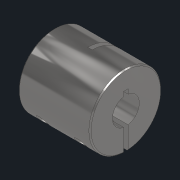
# Autodesk Inventor part: D_CPRC16-6-6
Saved by Autodesk Inventor 2022 (Build 260153000, 153)
## iProperties
Part Number: D_CPRC16-6-6
Material: 鋼、炭素鋼
Catalog Web Link: www.cadenas.de
Description: D_CPRC, CPRSC-Couplings - Rigid, Clamping Type
Vendor: MISUMI
Document SubType Name: Modeling
Designer: partserver
Manufacturer: MISUMI
Mass: 18.6575 g
Surface Area: 18.8292 cm^2
Volume: 2.37676 cm^3
Density: 7.85 g/cm^3
Appearance: 半つや出し
Category: PARTsolutions
Company: MISUMI
PSOL_IDENT_0: {$CADENAS_DATA\23d-libs\misumi\metric\50_couplings\parts\cprc.prj},182 {VTYP=3D},{NB=D_CPRC16-6-6},{
PSOL_IDENT_1: LINA=D_CPRC16-6-6},{NN=D_CPRC, CPRSC},{DATE=30.06.2021 13:25:02},{GEOMDATE=15.01.2008 11:35:00},{VER
PSOL_IDENT_2: SION=},{LINEID=10},{WBVAR=MAT,DD1,DD2},{WBNUMERIC=}  {NB=D_CPRC16-6-6},{LINA=D_CPRC16-6-6},{KT=DUMMY
PSOL_IDENT_3: },{PN=CPRC16-6-6},{MAT=1},{MATALG='1','Aluminium Alloy','2','Stainless Steel'},{ST=Alumite},{AC=Hex
PSOL_IDENT_4: Socket Head Cap Screw},{TYPE=CPRC},{D=16},{DD1=6},{DD1ALG1='5','5','6','6'},{DL=6},{DD2=6},{DD2ALG1='
PSOL_IDENT_5: 6','6'},{DR=6},{L=16},{M=2.5},{TSI=M2.5},{A=5},{A1=5.000},{TT=1},{TT1=1.000},{F=3.75},{TTT=1},{AT=0.
PSOL_IDENT_6: 3},{F1=3.750},{TSI1=4.800},{SC1=2.500},{SC2=5.970},{TSMD=2.500},{TSMIN=2.013},{L6=4.000}
NB: D_CPRC16-6-6
NN: D_CPRC, CPRSC
NT: Couplings - Rigid, Clamping Type
NBSYN: D_$TYPE.$D.-$DD1.-$DD2.
LINA: D_CPRC16-6-6
CATALOG: Misumi
PN: CPRC16-6-6
MAT: Aluminium Alloy
ST: Alumite
AC: Hex Socket Head Cap Screw
D: 16
DD1: 6
DD2: 6
L: 16
M: 2.5
A: 5
TT: 1
F: 3.75
SUPPLIER: MISUMI
ARTICLENO: D_CPRC16-6-6
BOMINFO: D_CPRC16-6-6
CREATOR: CADENAS GmbH
Title: D_CPRC16-6-6
Author: Cadenas PARTsolutions
Comments: Couplings - Rigid, Clamping Type
Autodesk Inventor part; units mm, degrees
sketch "Sketch_1" plane through (0, 0, 0) normal (0, 0, 1) x (1, 0, 0)
  line L0 (16, 0) -> (0, 0)
  line L1 (0, 3) -> (7.5, 3)
  line L2 (7.5, 3) -> (7.5, 3.1)
  line L3 (7.5, 3.1) -> (8.5, 3.1)
  line L4 (8.5, 3.1) -> (8.5, 3)
  line L5 (8.5, 3) -> (16, 3)
  line L6 (16, 3) -> (16, 7.75)
  line L7 (16, 7.75) -> (15.75, 8)
  line L8 (15.75, 8) -> (0.25, 8)
  line L9 (0.25, 8) -> (0, 7.75)
  line L10 (0, 7.75) -> (0, 3)
  constraints: 22 end point
revolve "Revolution1" add sketch "Sketch_1" angle 360 about axis through (16, 0, 0) along (1, 0, 0)
sketch "Sketch_2" plane through (0, 0, 0) normal (1, 0, 0) x (0, 1, 0)
  line L0 (0.5, 8) -> (-0.5, 8)
  line L1 (-0.5, 8) -> (-0.5, -4)
  line L2 (-0.5, -4) -> (0.5, -4)
  line L3 (0.5, -4) -> (0.5, 8)
  constraints: 8 end point
extrude "Extrusion1" cut sketch "Sketch_2" along normal blind 16
sketch "Sketch_3" plane through (0, 0, 0) normal (0, 1, 0) x (-1, 0, 0)
  line L0 (-8.5, 0) -> (-7.5, 0)
  line L1 (-7.5, 0) -> (-7.5, -8)
  line L2 (-7.5, -8) -> (-8.5, -8)
  line L3 (-8.5, -8) -> (-8.5, 0)
  line L4 (-8.5, 0) -> (-7.5, 0)
  constraints: 10 end point
revolve "Revolution2" cut sketch "Sketch_3" angle 180 about axis through (8.5, 0, 0) along (1, 0, 0)
sketch "Sketch_4" plane through (3.75, 0, 0) normal (1, 0, 0) x (0, 0, -1)
  line L0 (-5, 8) -> (-5, -8)
  line L1 (-5, -8) -> (-6.25, -8)
  line L2 (-6.25, -8) -> (-6.25, 2.5)
  line L3 (-6.25, 2.5) -> (-7.4, 2.5)
  line L4 (-7.4, 2.5) -> (-7.4, 8)
  line L5 (-7.4, 8) -> (-5, 8)
  line L6 (-5, 8) -> (-5, -8)
  constraints: 14 end point
revolve "Revolution3" cut sketch "Sketch_4" angle 360 about axis through (3.75, 8, 5) along (0, 1, 0)
sketch "Sketch_5" plane through (12.25, 0, 0) normal (1, 0, 0) x (0, 0, -1)
  line L0 (-5, 8) -> (-5, -8)
  line L1 (-5, -8) -> (-6.25, -8)
  line L2 (-6.25, -8) -> (-6.25, 2.5)
  line L3 (-6.25, 2.5) -> (-7.4, 2.5)
  line L4 (-7.4, 2.5) -> (-7.4, 8)
  line L5 (-7.4, 8) -> (-5, 8)
  line L6 (-5, 8) -> (-5, -8)
  constraints: 14 end point
revolve "Revolution4" cut sketch "Sketch_5" angle 360 about axis through (12.25, 8, 5) along (0, 1, 0)
ref_plane "L_XY" through (3.75, 2.5, 5) normal (0, 1, 0) x (1, 0, 0)
ref_plane "L_YZ" through (3.75, 2.5, 5) normal (1, 0, 0) x (0, 0, -1)
ref_plane "L_ZX" through (3.75, 2.5, 5) normal (0, 0, -1) x (0, 1, 0)
ref_plane "R_XY" through (12.25, 2.5, 5) normal (0, 1, 0) x (1, 0, 0)
ref_plane "R_YZ" through (12.25, 2.5, 5) normal (1, 0, 0) x (0, 0, -1)
ref_plane "R_ZX" through (12.25, 2.5, 5) normal (0, 0, -1) x (0, 1, 0)
body "Solid1"
